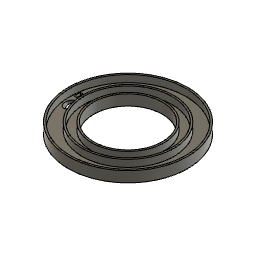
Neopixel Ring v5 (Autodesk Fusion 360 design; units mm, degrees)
Autodesk Fusion 360 part; units mm, degrees
sketch "Sketch1" plane through (0, 0, 0) normal (0, 1, 0) x (1, 0, 0)
  circle A0 centre (0, 0) radius 26
  circle A1 centre (0, 0) radius 32.875
  circle A2 centre (0, 0) radius 25
  circle A3 centre (0, 0) radius 33.875
  circle A4 centre (0, 0) radius 19.5
  circle A5 centre (0, 0) radius 20.5
  dimension "d1" = 67.75
  dimension "d2" = 50
  dimension "d3" = 52
  dimension "d4" = 65.75
  dimension "d10" = 39
  dimension "d25" = 41
  constraint coincident A0.centre A1.centre
  constraint concentric A0 A1
  constraint concentric A3 A4
  constraint concentric A1 A5
  measures "d1" diameter of A3
  measures "d2" diameter of A2
  measures "d3" diameter of A0
  measures "d4" diameter of A1
  measures "d10" diameter of A4
  measures "d25" diameter of A5
extrude "Extrude1" add sketch "Sketch1" along normal blind 2 contours A1 | A2 | A5 makes body 1 at (30.3641, 0, 2.925) makes body 2 at (23.0736, 0, 1.242)
extrude "Extrude2" add sketch "Sketch1" along normal blind 6 bodies 2 1
sketch "Sketch2" plane through (0, 2, 0) normal (0, 1, 0) x (-1, 0, 0)
  circle A0 centre (0, 0) radius 26
  circle A1 centre (0, 0) radius 32.875
  line L0 (32, -5) -> (30.5, -5)
  line L1 (30.5, -5) -> (30.5, -1.5)
  line L2 (30.5, -1.5) -> (32, -1.5)
  line L3 (32, -1.5) -> (32, -5)
  line L4 (26.2, -1.5) -> (27.7, -1.5)
  line L5 (27.7, -1.5) -> (27.7, -5)
  line L6 (27.7, -5) -> (26.2, -5)
  line L7 (26.2, -5) -> (26.2, -1.5)
  line L8 (32, 4) -> (26, 4)
  dimension "d13" = 1.5
  dimension "d14" = 3.5
  dimension "d15" = 1.5
  dimension "d16" = 3.5
  constraint horizontal L0
  constraint vertical L1
  constraint horizontal L2
  constraint vertical L3
  constraint horizontal L4
  constraint vertical L5
  constraint horizontal L6
  constraint vertical L7
  constraint horizontal L8
  measures "d13" distance of L0.start L0.end
  measures "d14" distance of L0.start L2.end
  measures "d15" distance of L4.start L4.end
  measures "d16" distance of L4.start L6.end
extrude "Extrude3" cut sketch "Sketch2" against normal blind 2 contours L0 L1 L2 L3 | L4 L5 L6 L7 bodies 2
ref_plane "WorkPlane1" through (-29, 2, 4) normal (0, 0.707107, 0.707107) x (1, 0, 0)
sketch "Sketch4" plane through (-29, 2, 4) normal (0, 0.707107, 0.707107) x (1, 0, 0)
  circle A0 centre (0, 0) radius 2.5
  dimension "d20" = 5
  constraint coincident A0.centre origin
  measures "d20" diameter of A0
extrude "Extrude4" cut sketch "Sketch4" along normal blind 10 and the other way blind 10 bodies 2
sketch "Sketch3" plane through (0, 2, 0) normal (0, 1, 0) x (-1, 0, 0)
  line L0 (30.5, -4) -> (30.5, -0.5)
  line L1 (30.5, -0.5) -> (32, -0.5)
  line L2 (32, -0.5) -> (32, -4)
  line L3 (32, -4) -> (30.5, -4)
  line L4 (27.7, -0.5) -> (27.7, -4)
  line L5 (27.7, -4) -> (26.2, -4)
  line L6 (26.2, -4) -> (26.2, -0.5)
  line L7 (26.2, -0.5) -> (27.7, -0.5)
  circle A0 centre (0, 0) radius 26
  circle A1 centre (0, 0) radius 33
